Autodesk Fusion 360 part; units mm, degrees
note: some values were not read from the file. Set by a fixed rule: which sketch regions a step uses.
(part 3 of 20)
  spline S10 degree 5 poles (-7.9771, -12.1359) (-7.9772, -12.1359) (-7.9772, -12.136) (-7.9774, -12.1362) (-7.9776, -12.1365) (-7.9779, -12.137) (-7.9782, -12.1375) (-7.9786, -12.1381) (-7.979, -12.1388) (-7.9794, -12.1395) (-7.9799, -12.1403) (-7.9804, -12.1411) (-7.981, -12.1421) (-7.9816, -12.1431) (-7.9823, -12.1441) (-7.9829, -12.1452) (-7.9836, -12.1464) (-7.9844, -12.1477) (-7.9852, -12.149) (-7.986, -12.1504) (-7.9868, -12.1518) (-7.9877, -12.1533) (-7.9886, -12.1549) (-7.9896, -12.1565) (-7.9905, -12.1582) (-7.9915, -12.16) (-7.9926, -12.1618) (-7.9936, -12.1637) (-7.9947, -12.1656) (-7.9958, -12.1676) (-7.997, -12.1696) (-7.9982, -12.1718) (-7.9994, -12.1739) (-8.0006, -12.1762) (-8.0018, -12.1785) (-8.0031, -12.1808) (-8.0044, -12.1832) (-8.0057, -12.1857) (-8.0071, -12.1882) (-8.0084, -12.1908) (-8.0098, -12.1934) (-8.0113, -12.1961) (-8.0127, -12.1988) (-8.0142, -12.2016) (-8.0156, -12.2045) (-8.0171, -12.2074) (-8.0187, -12.2104) (-8.0202, -12.2134) (-8.0218, -12.2164) (-8.0233, -12.2196) (-8.0249, -12.2228) (-8.0265, -12.226) (-8.0282, -12.2293) (-8.0298, -12.2326) (-8.0315, -12.236) (-8.0332, -12.2395) (-8.0349, -12.243) (-8.0366, -12.2465) (-8.0383, -12.2501) (-8.0401, -12.2538) (-8.0419, -12.2575) (-8.0436, -12.2612) (-8.0454, -12.265) (-8.0472, -12.2689) (-8.0491, -12.2728) (-8.0509, -12.2768) (-8.0527, -12.2808) (-8.0546, -12.2848) (-8.0565, -12.289) (-8.0584, -12.2931) (-8.0603, -12.2973) (-8.0622, -12.3016) (-8.0641, -12.3059) (-8.066, -12.3102) (-8.068, -12.3146) (-8.0699, -12.3191) (-8.0719, -12.3236) (-8.0739, -12.3281) (-8.0759, -12.3327) (-8.0779, -12.3374) (-8.0799, -12.3421) (-8.0819, -12.3468) (-8.0839, -12.3516) (-8.0859, -12.3564) (-8.088, -12.3613) (-8.09, -12.3662) (-8.0921, -12.3712) (-8.0941, -12.3762) (-8.0962, -12.3813) (-8.0983, -12.3864) (-8.1004, -12.3915) (-8.1025, -12.3967) (-8.1046, -12.402) (-8.1067, -12.4073) (-8.1088, -12.4126) (-8.1109, -12.418) (-8.113, -12.4234) (-8.1151, -12.4289) (-8.1173, -12.4344) (-8.1194, -12.4399) (-8.1215, -12.4455) (-8.1237, -12.4512) (-8.1258, -12.4568) (-8.128, -12.4626) (-8.1302, -12.4683) (-8.1323, -12.4742) (-8.1345, -12.48) (-8.1366, -12.4859) (-8.1388, -12.4919) (-8.141, -12.4979) (-8.1432, -12.5039) (-8.1453, -12.51) (-8.1475, -12.5161) (-8.1497, -12.5222) (-8.1519, -12.5284) (-8.1541, -12.5347) (-8.1563, -12.5409) (-8.1584, -12.5473) (-8.1606, -12.5536) (-8.1628, -12.56) (-8.165, -12.5665) (-8.1672, -12.5729) (-8.1694, -12.5795) (-8.1716, -12.586) (-8.1738, -12.5926) (-8.176, -12.5993) (-8.1782, -12.606) (-8.1803, -12.6127) (-8.1825, -12.6195) (-8.1847, -12.6263) (-8.1869, -12.6331) (-8.1891, -12.64) (-8.1913, -12.6469) (-8.1935, -12.6539) (-8.1956, -12.6609) (-8.1978, -12.6679) (-8.2, -12.675) (-8.2022, -12.6821) (-8.2044, -12.6893) (-8.2065, -12.6965) (-8.2087, -12.7037) (-8.2109, -12.711) (-8.213, -12.7183) (-8.2152, -12.7256) (-8.2173, -12.733) (-8.2195, -12.7404) (-8.2216, -12.7479) (-8.2238, -12.7554) (-8.2259, -12.7629) (-8.2281, -12.7705) (-8.2302, -12.7781) (-8.2323, -12.7857) (-8.2345, -12.7934) (-8.2366, -12.8011) (-8.2387, -12.8089) (-8.2408, -12.8167) (-8.2429, -12.8245) (-8.245, -12.8324) (-8.2471, -12.8403) (-8.2492, -12.8482) (-8.2513, -12.8562) (-8.2534, -12.8642) (-8.2554, -12.8722) (-8.2575, -12.8803) (-8.2596, -12.8884) (-8.2616, -12.8966) (-8.2637, -12.9048) (-8.2657, -12.913) (-8.2678, -12.9212) (-8.2698, -12.9295) (-8.2718, -12.9379) (-8.2738, -12.9462) (-8.2759, -12.9546) (-8.2779, -12.963) (-8.2799, -12.9715) (-8.2818, -12.98) (-8.2838, -12.9885) (-8.2858, -12.9971) (-8.2878, -13.0057) (-8.2897, -13.0143) (-8.2917, -13.023) (-8.2936, -13.0317) (-8.2956, -13.0404) (-8.2975, -13.0492) (-8.2994, -13.058) (-8.3013, -13.0668) (-8.3032, -13.0757) (-8.3051, -13.0846) (-8.307, -13.0935) (-8.3089, -13.1025) (-8.3107, -13.1115) (-8.3126, -13.1205) (-8.3145, -13.1296) (-8.3163, -13.1386) (-8.3181, -13.1478) (-8.3199, -13.1569) (-8.3218, -13.1661) (-8.3236, -13.1753) (-8.3254, -13.1846) (-8.3271, -13.1939) (-8.3289, -13.2032) (-8.3307, -13.2125) (-8.3324, -13.2219) (-8.3342, -13.2313) (-8.3359, -13.2408) (-8.3376, -13.2503) (-8.3393, -13.2598) (-8.341, -13.2693) (-8.3427, -13.2789) (-8.3444, -13.2885) (-8.3461, -13.2981) (-8.3477, -13.3078) (-8.3494, -13.3174) (-8.351, -13.3272) (-8.3526, -13.3369) (-8.3542, -13.3467) (-8.3558, -13.3565) (-8.3574, -13.3663) (-8.359, -13.3762) (-8.3606, -13.3861) (-8.3621, -13.396) (-8.3637, -13.406) (-8.3652, -13.416) (-8.3667, -13.426) (-8.3682, -13.4361) (-8.3697, -13.4461) (-8.3712, -13.4563) (-8.3726, -13.4664) (-8.3741, -13.4766) (-8.3755, -13.4867) (-8.377, -13.497) (-8.3784, -13.5072) (-8.3798, -13.5175) (-8.3812, -13.5278) (-8.3826, -13.5382) (-8.3839, -13.5485) (-8.3853, -13.5589) (-8.3866, -13.5693) (-8.3879, -13.5798) (-8.3893, -13.5903) (-8.3906, -13.6008) (-8.3916, -13.6092) (-8.3924, -13.6155) (-8.3929, -13.6198) (-8.3931, -13.6219) knots 0 0 0 0 0 0 0.00416667 0.00833333 0.0125 0.01666667 0.02083333 0.025 0.02916667 0.03333333 0.0375 0.04166667 0.04583333 0.05 0.05416667 0.05833333 0.0625 0.06666667 0.07083333 0.075 0.07916667 0.08333333 0.0875 0.09166667 0.09583333 0.1 0.10416667 0.10833333 0.1125 0.11666667 0.12083333 0.125 0.12916667 0.13333333 0.1375 0.14166667 0.14583333 0.15 0.15416667 0.15833333 0.1625 0.16666667 0.17083333 0.175 0.17916667 0.18333333 0.1875 0.19166667 0.19583333 0.2 0.20416667 0.20833333 0.2125 0.21666667 0.22083333 0.225 0.22916667 0.23333333 0.2375 0.24166667 0.24583333 0.25 0.25416667 0.25833333 0.2625 0.26666667 0.27083333 0.275 0.27916667 0.28333333 0.2875 0.29166667 0.29583333 0.3 0.30416667 0.30833333 0.3125 0.31666667 0.32083333 0.325 0.32916667 0.33333333 0.3375 0.34166667 0.34583333 0.35 0.35416667 0.35833333 0.3625 0.36666667 0.37083333 0.375 0.37916667 0.38333333 0.3875 0.39166667 0.39583333 0.4 0.40416667 0.40833333 0.4125 0.41666667 0.42083333 0.425 0.42916667 0.43333333 0.4375 0.44166667 0.44583333 0.45 0.45416667 0.45833333 0.4625 0.46666667 0.47083333 0.475 0.47916667 0.48333333 0.4875 0.49166667 0.49583333 0.5 0.50416667 0.50833333 0.5125 0.51666667 0.52083333 0.525 0.52916667 0.53333333 0.5375 0.54166667 0.54583333 0.55 0.55416667 0.55833333 0.5625 0.56666667 0.57083333 0.575 0.57916667 0.58333333 0.5875 0.59166667 0.59583333 0.6 0.60416667 0.60833333 0.6125 0.61666667 0.62083333 0.625 0.62916667 0.63333333 0.6375 0.64166667 0.64583333 0.65 0.65416667 0.65833333 0.6625 0.66666667 0.67083333 0.675 0.67916667 0.68333333 0.6875 0.69166667 0.69583333 0.7 0.70416667 0.70833333 0.7125 0.71666667 0.72083333 0.725 0.72916667 0.73333333 0.7375 0.74166667 0.74583333 0.75 0.75416667 0.75833333 0.7625 0.76666667 0.77083333 0.775 0.77916667 0.78333333 0.7875 0.79166667 0.79583333 0.8 0.80416667 0.80833333 0.8125 0.81666667 0.82083333 0.825 0.82916667 0.83333333 0.8375 0.84166667 0.84583333 0.85 0.85416667 0.85833333 0.8625 0.86666667 0.87083333 0.875 0.87916667 0.88333333 0.8875 0.89166667 0.89583333 0.9 0.90416667 0.90833333 0.9125 0.91666667 0.92083333 0.925 0.92916667 0.93333333 0.9375 0.94166667 0.94583333 0.95 0.95416667 0.95833333 0.9625 0.96666667 0.97083333 0.975 0.97916667 0.98333333 0.9875 0.99166667 0.99583333 1 1 1 1 1 1
  arc A11 (-8.3931, -13.6219) -> (-7.6003, -14.0796) centre (0, 0) ccw
  spline S11 degree 5 poles (-7.6003, -14.0796) (-7.5986, -14.0783) (-7.5952, -14.0758) (-7.5901, -14.0719) (-7.5833, -14.0668) (-7.5749, -14.0604) (-7.5665, -14.0541) (-7.5581, -14.0477) (-7.5497, -14.0413) (-7.5414, -14.035) (-7.5331, -14.0286) (-7.5248, -14.0222) (-7.5166, -14.0159) (-7.5084, -14.0095) (-7.5002, -14.0032) (-7.4921, -13.9968) (-7.484, -13.9905) (-7.4759, -13.9841) (-7.4679, -13.9778) (-7.4599, -13.9714) (-7.4519, -13.9651) (-7.4439, -13.9588) (-7.436, -13.9525) (-7.4281, -13.9461) (-7.4203, -13.9398) (-7.4124, -13.9335) (-7.4046, -13.9272) (-7.3969, -13.9209) (-7.3892, -13.9146) (-7.3815, -13.9083) (-7.3738, -13.902) (-7.3662, -13.8958) (-7.3586, -13.8895) (-7.351, -13.8832) (-7.3435, -13.8769) (-7.336, -13.8707) (-7.3285, -13.8644) (-7.321, -13.8582) (-7.3136, -13.8519) (-7.3063, -13.8457) (-7.2989, -13.8395) (-7.2916, -13.8333) (-7.2843, -13.827) (-7.2771, -13.8208) (-7.2699, -13.8146) (-7.2627, -13.8084) (-7.2555, -13.8023) (-7.2484, -13.7961) (-7.2413, -13.7899) (-7.2343, -13.7837) (-7.2272, -13.7776) (-7.2203, -13.7714) (-7.2133, -13.7653) (-7.2064, -13.7592) (-7.1995, -13.753) (-7.1926, -13.7469) (-7.1858, -13.7408) (-7.179, -13.7347) (-7.1723, -13.7286) (-7.1655, -13.7226) (-7.1588, -13.7165) (-7.1522, -13.7104) (-7.1455, -13.7044) (-7.1389, -13.6983) (-7.1324, -13.6923) (-7.1259, -13.6863) (-7.1194, -13.6803) (-7.1129, -13.6743) (-7.1065, -13.6683) (-7.1001, -13.6623) (-7.0937, -13.6563) (-7.0874, -13.6504) (-7.0811, -13.6444) (-7.0748, -13.6385) (-7.0686, -13.6325) (-7.0624, -13.6266) (-7.0562, -13.6207) (-7.0501, -13.6148) (-7.044, -13.6089) (-7.0379, -13.6031) (-7.0319, -13.5972) (-7.0259, -13.5914) (-7.02, -13.5855) (-7.014, -13.5797) (-7.0081, -13.5739) (-7.0023, -13.5681) (-6.9965, -13.5624) (-6.9907, -13.5566) (-6.9849, -13.5508) (-6.9792, -13.5451) (-6.9735, -13.5394) (-6.9678, -13.5337) (-6.9622, -13.528) (-6.9566, -13.5223) (-6.9511, -13.5166) (-6.9455, -13.511) (-6.94, -13.5053) (-6.9346, -13.4997) (-6.9292, -13.4941) (-6.9238, -13.4885) (-6.9184, -13.4829) (-6.9131, -13.4774) (-6.9078, -13.4718) (-6.9026, -13.4663) (-6.8974, -13.4608) (-6.8922, -13.4553) (-6.8871, -13.4498) (-6.8819, -13.4444) (-6.8769, -13.4389) (-6.8718, -13.4335) (-6.8668, -13.4281) (-6.8618, -13.4227) (-6.8569, -13.4173) (-6.852, -13.412) (-6.8471, -13.4066) (-6.8423, -13.4013) (-6.8375, -13.396) (-6.8327, -13.3907) (-6.828, -13.3855) (-6.8233, -13.3802) (-6.8187, -13.375) (-6.814, -13.3698) (-6.8094, -13.3646) (-6.8049, -13.3595) (-6.8004, -13.3543) (-6.7959, -13.3492) (-6.7914, -13.3441) (-6.787, -13.339) (-6.7826, -13.334) (-6.7783, -13.329) (-6.774, -13.3239) (-6.7697, -13.319) (-6.7655, -13.314) (-6.7613, -13.309) (-6.7571, -13.3041) (-6.753, -13.2992) (-6.7489, -13.2944) (-6.7448, -13.2895) (-6.7408, -13.2847) (-6.7368, -13.2799) (-6.7328, -13.2751) (-6.7289, -13.2703) (-6.725, -13.2656) (-6.7212, -13.2609) (-6.7174, -13.2562) (-6.7136, -13.2516) (-6.7098, -13.2469) (-6.7061, -13.2423) (-6.7025, -13.2378) (-6.6988, -13.2332) (-6.6952, -13.2287) (-6.6917, -13.2242) (-6.6881, -13.2197) (-6.6846, -13.2153) (-6.6812, -13.2109) (-6.6778, -13.2065) (-6.6744, -13.2022) (-6.671, -13.1978) (-6.6677, -13.1935) (-6.6644, -13.1893) (-6.6612, -13.185) (-6.658, -13.1808) (-6.6548, -13.1767) (-6.6517, -13.1725) (-6.6486, -13.1684) (-6.6455, -13.1643) (-6.6425, -13.1603) (-6.6395, -13.1563) (-6.6366, -13.1523) (-6.6337, -13.1483) (-6.6308, -13.1444) (-6.628, -13.1405) (-6.6252, -13.1367) (-6.6224, -13.1328) (-6.6197, -13.1291) (-6.617, -13.1253) (-6.6143, -13.1216) (-6.6117, -13.1179) (-6.6091, -13.1143) (-6.6065, -13.1107) (-6.604, -13.1071) (-6.6016, -13.1036) (-6.5991, -13.1001) (-6.5967, -13.0966) (-6.5944, -13.0932) (-6.592, -13.0898) (-6.5897, -13.0865) (-6.5875, -13.0832) (-6.5853, -13.0799) (-6.5831, -13.0767) (-6.581, -13.0735) (-6.5788, -13.0703) (-6.5768, -13.0672) (-6.5747, -13.0642) (-6.5728, -13.0612) (-6.5708, -13.0582) (-6.5689, -13.0553) (-6.567, -13.0524) (-6.5651, -13.0495) (-6.5633, -13.0467) (-6.5616, -13.044) (-6.5598, -13.0413) (-6.5581, -13.0386) (-6.5565, -13.036) (-6.5549, -13.0334) (-6.5533, -13.0309) (-6.5517, -13.0284) (-6.5502, -13.026) (-6.5488, -13.0236) (-6.5473, -13.0213) (-6.5459, -13.019) (-6.5446, -13.0168) (-6.5433, -13.0146) (-6.542, -13.0125) (-6.5407, -13.0104) (-6.5395, -13.0084) (-6.5384, -13.0064) (-6.5372, -13.0045) (-6.5361, -13.0027) (-6.5351, -13.0009) (-6.5341, -12.9991) (-6.5331, -12.9974) (-6.5321, -12.9958) (-6.5312, -12.9942) (-6.5304, -12.9927) (-6.5295, -12.9913) (-6.5288, -12.9899) (-6.528, -12.9885) (-6.5273, -12.9873) (-6.5266, -12.986) (-6.526, -12.9849) (-6.5254, -12.9838) (-6.5248, -12.9828) (-6.5243, -12.9818) (-6.5238, -12.9809) (-6.5234, -12.9801) (-6.523, -12.9794) (-6.5226, -12.9787) (-6.5223, -12.9781) (-6.522, -12.9775) (-6.5218, -12.977) (-6.5216, -12.9767) (-6.5215, -12.9765) (-6.5214, -12.9764) (-6.5214, -12.9763) knots -1 -1 -1 -1 -1 -1 -0.99583333 -0.99166667 -0.9875 -0.98333333 -0.97916667 -0.975 -0.97083333 -0.96666667 -0.9625 -0.95833333 -0.95416667 -0.95 -0.94583333 -0.94166667 -0.9375 -0.93333333 -0.92916667 -0.925 -0.92083333 -0.91666667 -0.9125 -0.90833333 -0.90416667 -0.9 -0.89583333 -0.89166667 -0.8875 -0.88333333 -0.87916667 -0.875 -0.87083333 -0.86666667 -0.8625 -0.85833333 -0.85416667 -0.85 -0.84583333 -0.84166667 -0.8375 -0.83333333 -0.82916667 -0.825 -0.82083333 -0.81666667 -0.8125 -0.80833333 -0.80416667 -0.8 -0.79583333 -0.79166667 -0.7875 -0.78333333 -0.77916667 -0.775 -0.77083333 -0.76666667 -0.7625 -0.75833333 -0.75416667 -0.75 -0.74583333 -0.74166667 -0.7375 -0.73333333 -0.72916667 -0.725 -0.72083333 -0.71666667 -0.7125 -0.70833333 -0.70416667 -0.7 -0.69583333 -0.69166667 -0.6875 -0.68333333 -0.67916667 -0.675 -0.67083333 -0.66666667 -0.6625 -0.65833333 -0.65416667 -0.65 -0.64583333 -0.64166667 -0.6375 -0.63333333 -0.62916667 -0.625 -0.62083333 -0.61666667 -0.6125 -0.60833333 -0.60416667 -0.6 -0.59583333 -0.59166667 -0.5875 -0.58333333 -0.57916667 -0.575 -0.57083333 -0.56666667 -0.5625 -0.55833333 -0.55416667 -0.55 -0.54583333 -0.54166667 -0.5375 -0.53333333 -0.52916667 -0.525 -0.52083333 -0.51666667 -0.5125 -0.50833333 -0.50416667 -0.5 -0.49583333 -0.49166667 -0.4875 -0.48333333 -0.47916667 -0.475 -0.47083333 -0.46666667 -0.4625 -0.45833333 -0.45416667 -0.45 -0.44583333 -0.44166667 -0.4375 -0.43333333 -0.42916667 -0.425 -0.42083333 -0.41666667 -0.4125 -0.40833333 -0.40416667 -0.4 -0.39583333 -0.39166667 -0.3875 -0.38333333 -0.37916667 -0.375 -0.37083333 -0.36666667 -0.3625 -0.35833333 -0.35416667 -0.35 -0.34583333 -0.34166667 -0.3375 -0.33333333 -0.32916667 -0.325 -0.32083333 -0.31666667 -0.3125 -0.30833333 -0.30416667 -0.3 -0.29583333 -0.29166667 -0.2875 -0.28333333 -0.27916667 -0.275 -0.27083333 -0.26666667 -0.2625 -0.25833333 -0.25416667 -0.25 -0.24583333 -0.24166667 -0.2375 -0.23333333 -0.22916667 -0.225 -0.22083333 -0.21666667 -0.2125 -0.20833333 -0.20416667 -0.2 -0.19583333 -0.19166667 -0.1875 -0.18333333 -0.17916667 -0.175 -0.17083333 -0.16666667 -0.1625 -0.15833333 -0.15416667 -0.15 -0.14583333 -0.14166667 -0.1375 -0.13333333 -0.12916667 -0.125 -0.12083333 -0.11666667 -0.1125 -0.10833333 -0.10416667 -0.1 -0.09583333 -0.09166667 -0.0875 -0.08333333 -0.07916667 -0.075 -0.07083333 -0.06666667 -0.0625 -0.05833333 -0.05416667 -0.05 -0.04583333 -0.04166667 -0.0375 -0.03333333 -0.02916667 -0.025 -0.02083333 -0.01666667 -0.0125 -0.00833333 -0.00416667 0 0 0 0 0 0
  line L22 (-6.5214, -12.9763) -> (-6.5211, -12.9757)
  line L23 (-6.5211, -12.9757) -> (-6.1743, -12.2858)
  arc A12 (-6.1743, -12.2858) -> (-4.9987, -12.8092) centre (0, 0) ccw
  line L24 (-4.9987, -12.8092) -> (-5.2794, -13.5286)
  line L25 (-5.2794, -13.5286) -> (-5.2796, -13.5292)
  spline S12 degree 5 poles (-5.2796, -13.5292) (-5.2796, -13.5293) (-5.2797, -13.5294) (-5.2798, -13.5296) (-5.2799, -13.53) (-5.2801, -13.5305) (-5.2803, -13.531) (-5.2805, -13.5317) (-5.2808, -13.5324) (-5.2811, -13.5332) (-5.2814, -13.5341) (-5.2818, -13.5351) (-5.2821, -13.5361) (-5.2825, -13.5372) (-5.2829, -13.5383) (-5.2833, -13.5396) (-5.2838, -13.5409) (-5.2843, -13.5423) (-5.2848, -13.5437) (-5.2853, -13.5452) (-5.2858, -13.5468) (-5.2863, -13.5485) (-5.2869, -13.5502) (-5.2875, -13.552) (-5.2881, -13.5539) (-5.2887, -13.5558) (-5.2893, -13.5578) (-5.29, -13.5598) (-5.2907, -13.5619) (-5.2913, -13.5641) (-5.292, -13.5664) (-5.2927, -13.5687) (-5.2935, -13.5711) (-5.2942, -13.5735) (-5.2949, -13.576) (-5.2957, -13.5786) (-5.2965, -13.5812) (-5.2972, -13.5839) (-5.298, -13.5866) (-5.2988, -13.5894) (-5.2997, -13.5923) (-5.3005, -13.5952) (-5.3013, -13.5982) (-5.3022, -13.6012) (-5.303, -13.6043) (-5.3039, -13.6075) (-5.3047, -13.6107) (-5.3056, -13.614) (-5.3065, -13.6173) (-5.3074, -13.6207) (-5.3083, -13.6241) (-5.3092, -13.6276) (-5.3101, -13.6312) (-5.3111, -13.6348) (-5.312, -13.6385) (-5.3129, -13.6422) (-5.3138, -13.646) (-5.3148, -13.6498) (-5.3157, -13.6537) (-5.3167, -13.6576) (-5.3176, -13.6616) (-5.3186, -13.6657) (-5.3196, -13.6698) (-5.3205, -13.6739) (-5.3215, -13.6781) (-5.3225, -13.6824) (-5.3235, -13.6867) (-5.3244, -13.691) (-5.3254, -13.6954) (-5.3264, -13.6999) (-5.3274, -13.7044) (-5.3284, -13.709) (-5.3293, -13.7136) (-5.3303, -13.7183) (-5.3313, -13.723) (-5.3323, -13.7277) (-5.3333, -13.7325) (-5.3343, -13.7374) (-5.3353, -13.7423) (-5.3363, -13.7473) (-5.3372, -13.7523) (-5.3382, -13.7573) (-5.3392, -13.7624) (-5.3402, -13.7676) (-5.3412, -13.7728) (-5.3422, -13.778) (-5.3431, -13.7833) (-5.3441, -13.7886) (-5.3451, -13.794) (-5.3461, -13.7994) (-5.347, -13.8049) (-5.348, -13.8104) (-5.3489, -13.816) (-5.3499, -13.8216) (-5.3509, -13.8273) (-5.3518, -13.833) (-5.3528, -13.8387) (-5.3537, -13.8445) (-5.3546, -13.8503) (-5.3556, -13.8562) (-5.3565, -13.8621) (-5.3574, -13.8681) (-5.3583, -13.8741) (-5.3593, -13.8801) (-5.3602, -13.8862) (-5.3611, -13.8924) (-5.362, -13.8986) (-5.3629, -13.9048) (-5.3638, -13.911) (-5.3646, -13.9173) (-5.3655, -13.9237) (-5.3664, -13.9301) (-5.3672, -13.9365) (-5.3681, -13.943) (-5.3689, -13.9495) (-5.3698, -13.9561) (-5.3706, -13.9627) (-5.3714, -13.9693) (-5.3723, -13.976) (-5.3731, -13.9827) (-5.3739, -13.9895) (-5.3747, -13.9963) (-5.3755, -14.0031) (-5.3762, -14.01) (-5.377, -14.0169) (-5.3778, -14.0238) (-5.3785, -14.0308) (-5.3793, -14.0379) (-5.38, -14.0449) (-5.3807, -14.0521) (-5.3814, -14.0592) (-5.3821, -14.0664) (-5.3828, -14.0736) (-5.3835, -14.0809) (-5.3842, -14.0882) (-5.3849, -14.0955) (-5.3855, -14.1029) (-5.3862, -14.1103) (-5.3868, -14.1178) (-5.3874, -14.1253) (-5.3881, -14.1328) (-5.3887, -14.1403) (-5.3893, -14.1479) (-5.3899, -14.1556) (-5.3904, -14.1632) (-5.391, -14.171) (-5.3915, -14.1787) (-5.3921, -14.1865) (-5.3926, -14.1943) (-5.3931, -14.2021) (-5.3936, -14.21) (-5.3941, -14.2179) (-5.3946, -14.2259) (-5.3951, -14.2339) (-5.3955, -14.2419) (-5.396, -14.25) (-5.3964, -14.2581) (-5.3968, -14.2662) (-5.3973, -14.2744) (-5.3976, -14.2826) (-5.398, -14.2908) (-5.3984, -14.2991) (-5.3988, -14.3074) (-5.3991, -14.3157) (-5.3994, -14.3241) (-5.3998, -14.3325) (-5.4001, -14.3409) (-5.4003, -14.3493) (-5.4006, -14.3578) (-5.4009, -14.3664) (-5.4011, -14.3749) (-5.4014, -14.3835) (-5.4016, -14.3922) (-5.4018, -14.4008) (-5.402, -14.4095) (-5.4022, -14.4182) (-5.4023, -14.427) (-5.4025, -14.4358) (-5.4026, -14.4446) (-5.4028, -14.4535) (-5.4029, -14.4623) (-5.403, -14.4712) (-5.403, -14.4802) (-5.4031, -14.4892) (-5.4031, -14.4982) (-5.4032, -14.5072) (-5.4032, -14.5163) (-5.4032, -14.5254) (-5.4032, -14.5345) (-5.4032, -14.5437) (-5.4031, -14.5528) (-5.4031, -14.5621) (-5.403, -14.5713) (-5.4029, -14.5806) (-5.4028, -14.5899) (-5.4027, -14.5992) (-5.4025, -14.6086) (-5.4024, -14.618) (-5.4022, -14.6274) (-5.402, -14.6369) (-5.4018, -14.6464) (-5.4016, -14.6559) (-5.4013, -14.6654) (-5.4011, -14.675) (-5.4008, -14.6846) (-5.4005, -14.6942) (-5.4002, -14.7038) (-5.3999, -14.7135) (-5.3996, -14.7232) (-5.3992, -14.733) (-5.3988, -14.7427) (-5.3985, -14.7525) (-5.3981, -14.7624) (-5.3976, -14.7722) (-5.3972, -14.7821) (-5.3967, -14.792) (-5.3963, -14.8019) (-5.3958, -14.8119) (-5.3953, -14.8218) (-5.3947, -14.8319) (-5.3942, -14.8419) (-5.3936, -14.852) (-5.393, -14.862) (-5.3924, -14.8722) (-5.3918, -14.8823) (-5.3912, -14.8925) (-5.3905, -14.9027) (-5.3899, -14.9129) (-5.3892, -14.9231) (-5.3885, -14.9334) (-5.3877, -14.9437) (-5.387, -14.954) (-5.3862, -14.9644) (-5.3854, -14.9747) (-5.3846, -14.9851) (-5.3838, -14.9956) (-5.383, -15.006) (-5.3821, -15.0165) (-5.3813, -15.027) (-5.3804, -15.0375) (-5.3794, -15.0481) (-5.3787, -15.0565) (-5.3781, -15.0629) (-5.3777, -15.0671) (-5.3776, -15.0692) knots 0 0 0 0 0 0 0.00416667 0.00833333 0.0125 0.01666667 0.02083333 0.025 0.02916667 0.03333333 0.0375 0.04166667 0.04583333 0.05 0.05416667 0.05833333 0.0625 0.06666667 0.07083333 0.075 0.07916667 0.08333333 0.0875 0.09166667 0.09583333 0.1 0.10416667 0.10833333 0.1125 0.11666667 0.12083333 0.125 0.12916667 0.13333333 0.1375 0.14166667 0.14583333 0.15 0.15416667 0.15833333 0.1625 0.16666667 0.17083333 0.175 0.17916667 0.18333333 0.1875 0.19166667 0.19583333 0.2 0.20416667 0.20833333 0.2125 0.21666667 0.22083333 0.225 0.22916667 0.23333333 0.2375 0.24166667 0.24583333 0.25 0.25416667 0.25833333 0.2625 0.26666667 0.27083333 0.275 0.27916667 0.28333333 0.2875 0.29166667 0.29583333 0.3 0.30416667 0.30833333 0.3125 0.31666667 0.32083333 0.325 0.32916667 0.33333333 0.3375 0.34166667 0.34583333 0.35 0.35416667 0.35833333 0.3625 0.36666667 0.37083333 0.375 0.37916667 0.38333333 0.3875 0.39166667 0.39583333 0.4 0.40416667 0.40833333 0.4125 0.41666667 0.42083333 0.425 0.42916667 0.43333333 0.4375 0.44166667 0.44583333 0.45 0.45416667 0.45833333 0.4625 0.46666667 0.47083333 0.475 0.47916667 0.48333333 0.4875 0.49166667 0.49583333 0.5 0.50416667 0.50833333 0.5125 0.51666667 0.52083333 0.525 0.52916667 0.53333333 0.5375 0.54166667 0.54583333 0.55 0.55416667 0.55833333 0.5625 0.56666667 0.57083333 0.575 0.57916667 0.58333333 0.5875 0.59166667 0.59583333 0.6 0.60416667 0.60833333 0.6125 0.61666667 0.62083333 0.625 0.62916667 0.63333333 0.6375 0.64166667 0.64583333 0.65 0.65416667 0.65833333 0.6625 0.66666667 0.67083333 0.675 0.67916667 0.68333333 0.6875 0.69166667 0.69583333 0.7 0.70416667 0.70833333 0.7125 0.71666667 0.72083333 0.725 0.72916667 0.73333333 0.7375 0.74166667 0.74583333 0.75 0.75416667 0.75833333 0.7625 0.76666667 0.77083333 0.775 0.77916667 0.78333333 0.7875 0.79166667 0.79583333 0.8 0.80416667 0.80833333 0.8125 0.81666667 0.82083333 0.825 0.82916667 0.83333333 0.8375 0.84166667 0.84583333 0.85 0.85416667 0.85833333 0.8625 0.86666667 0.87083333 0.875 0.87916667 0.88333333 0.8875 0.89166667 0.89583333 0.9 0.90416667 0.90833333 0.9125 0.91666667 0.92083333 0.925 0.92916667 0.93333333 0.9375 0.94166667 0.94583333 0.95 0.95416667 0.95833333 0.9625 0.96666667 0.97083333 0.975 0.97916667 0.98333333 0.9875 0.99166667 0.99583333 1 1 1 1 1 1
  arc A13 (-5.3776, -15.0692) -> (-4.5069, -15.3521) centre (0, 0) ccw
  spline S13 degree 5 poles (-4.5069, -15.3521) (-4.5055, -15.3505) (-4.5027, -15.3473) (-4.4985, -15.3425) (-4.493, -15.3361) (-4.486, -15.3281) (-4.4791, -15.3201) (-4.4722, -15.3121) (-4.4654, -15.3042) (-4.4586, -15.2962) (-4.4518, -15.2883) (-4.445, -15.2803) (-4.4383, -15.2724) (-4.4316, -15.2645) (-4.4249, -15.2565) (-4.4183, -15.2486) (-4.4117, -15.2407) (-4.4051, -15.2329) (-4.3985, -15.225) (-4.392, -15.2171) (-4.3855, -15.2093) (-4.3791, -15.2014) (-4.3726, -15.1936) (-4.3662, -15.1858) (-4.3599, -15.178) (-4.3535, -15.1702) (-4.3472, -15.1624) (-4.3409, -15.1546) (-4.3347, -15.1468) (-4.3285, -15.1391) (-4.3223, -15.1313) (-4.3161, -15.1236) (-4.31, -15.1159) (-4.3039, -15.1082) (-4.2978, -15.1005) (-4.2918, -15.0928) (-4.2858, -15.0851) (-4.2798, -15.0775) (-4.2738, -15.0698) (-4.2679, -15.0622) (-4.262, -15.0546) (-4.2562, -15.047) (-4.2503, -15.0394) (-4.2445, -15.0318) (-4.2388, -15.0242) (-4.233, -15.0167) (-4.2273, -15.0092) (-4.2216, -15.0016) (-4.216, -14.9941) (-4.2104, -14.9866) (-4.2048, -14.9791) (-4.1992, -14.9717) (-4.1937, -14.9642) (-4.1882, -14.9568) (-4.1827, -14.9494) (-4.1773, -14.942) (-4.1719, -14.9346) (-4.1665, -14.9272) (-4.1612, -14.9198) (-4.1559, -14.9125) (-4.1506, -14.9052) (-4.1453, -14.8978) (-4.1401, -14.8905) (-4.1349, -14.8833) (-4.1297, -14.876) (-4.1246, -14.8687) (-4.1195, -14.8615) (-4.1144, -14.8543) (-4.1094, -14.8471) (-4.1044, -14.8399) (-4.0994, -14.8328) (-4.0944, -14.8256) (-4.0895, -14.8185) (-4.0846, -14.8114) (-4.0798, -14.8043) (-4.0749, -14.7972) (-4.0701, -14.7901) (-4.0654, -14.7831) (-4.0606, -14.7761) (-4.0559, -14.7691) (-4.0512, -14.7621) (-4.0466, -14.7551) (-4.042, -14.7482) (-4.0374, -14.7413) (-4.0328, -14.7344) (-4.0283, -14.7275) (-4.0238, -14.7206) (-4.0193, -14.7138) (-4.0149, -14.707) (-4.0105, -14.7002) (-4.0061, -14.6934) (-4.0018, -14.6866) (-3.9974, -14.6799) (-3.9932, -14.6731) (-3.9889, -14.6665) (-3.9847, -14.6598) (-3.9805, -14.6531) (-3.9763, -14.6465) (-3.9722, -14.6399) (-3.9681, -14.6333) (-3.964, -14.6267) (-3.96, -14.6202) (-3.9559, -14.6137) (-3.952, -14.6072) (-3.948, -14.6007) (-3.9441, -14.5942) (-3.9402, -14.5878) (-3.9363, -14.5814) (-3.9325, -14.575) (-3.9287, -14.5687) (-3.9249, -14.5623) (-3.9212, -14.556) (-3.9175, -14.5497) (-3.9138, -14.5435) (-3.9101, -14.5373) (-3.9065, -14.5311) (-3.9029, -14.5249) (-3.8993, -14.5187) (-3.8958, -14.5126) (-3.8923, -14.5065) (-3.8888, -14.5004) (-3.8854, -14.4944) (-3.882, -14.4883) (-3.8786, -14.4824) (-3.8752, -14.4764) (-3.8719, -14.4704) (-3.8686, -14.4645) (-3.8654, -14.4587) (-3.8621, -14.4528) (-3.8589, -14.447) (-3.8558, -14.4412) (-3.8526, -14.4354) (-3.8495, -14.4297) (-3.8464, -14.424) (-3.8434, -14.4183) (-3.8403, -14.4126) (-3.8373, -14.407) (-3.8344, -14.4014) (-3.8314, -14.3959) (-3.8285, -14.3903) (-3.8257, -14.3848) (-3.8228, -14.3794) (-3.82, -14.3739) (-3.8172, -14.3685) (-3.8144, -14.3632) (-3.8117, -14.3578) (-3.809, -14.3525) (-3.8063, -14.3473) (-3.8037, -14.342) (-3.8011, -14.3368) (-3.7985, -14.3316) (-3.796, -14.3265) (-3.7934, -14.3214) (-3.791, -14.3163) (-3.7885, -14.3113) (-3.7861, -14.3063) (-3.7836, -14.3013) (-3.7813, -14.2964) (-3.7789, -14.2915) (-3.7766, -14.2867) (-3.7743, -14.2819) (-3.7721, -14.2771) (-3.7698, -14.2723) (-3.7676, -14.2676) (-3.7655, -14.263) (-3.7633, -14.2583) (-3.7612, -14.2537) (-3.7591, -14.2492) (-3.7571, -14.2447) (-3.755, -14.2402) (-3.753, -14.2358) (-3.7511, -14.2314) (-3.7491, -14.227) (-3.7472, -14.2227) (-3.7453, -14.2185) (-3.7435, -14.2142) (-3.7416, -14.21) (-3.7398, -14.2059) (-3.7381, -14.2018) (-3.7363, -14.1977) (-3.7346, -14.1937) (-3.7329, -14.1898) (-3.7313, -14.1858) (-3.7296, -14.1819) (-3.728, -14.1781) (-3.7265, -14.1743) (-3.7249, -14.1706) (-3.7234, -14.1669) (-3.7219, -14.1632) (-3.7204, -14.1596) (-3.719, -14.1561) (-3.7176, -14.1525) (-3.7162, -14.1491) (-3.7149, -14.1457) (-3.7136, -14.1423) (-3.7123, -14.139) (-3.711, -14.1357) (-3.7097, -14.1325) (-3.7085, -14.1293) (-3.7073, -14.1262) (-3.7062, -14.1232) (-3.7051, -14.1202) (-3.704, -14.1172) (-3.7029, -14.1143) (-3.7018, -14.1114) (-3.7008, -14.1086) (-3.6998, -14.1059) (-3.6988, -14.1032) (-3.6979, -14.1006) (-3.697, -14.098) (-3.6961, -14.0955) (-3.6952, -14.093) (-3.6944, -14.0906) (-3.6936, -14.0883) (-3.6928, -14.086) (-3.692, -14.0838) (-3.6913, -14.0816) (-3.6906, -14.0795) (-3.6899, -14.0775) (-3.6892, -14.0755) (-3.6886, -14.0736) (-3.688, -14.0717) (-3.6874, -14.0699) (-3.6869, -14.0682) (-3.6863, -14.0665) (-3.6858, -14.0649) (-3.6853, -14.0634) (-3.6849, -14.0619) (-3.6845, -14.0606) (-3.6841, -14.0592) (-3.6837, -14.058) (-3.6833, -14.0568) (-3.683, -14.0557) (-3.6827, -14.0546) (-3.6824, -14.0537) (-3.6821, -14.0528) (-3.6819, -14.0519) (-3.6817, -14.0512) (-3.6815, -14.0505) (-3.6813, -14.0499) (-3.6812, -14.0494) (-3.6811, -14.0491) (-3.681, -14.0488) (-3.681, -14.0487) (-3.681, -14.0486) knots -1 -1 -1 -1 -1 -1 -0.99583333 -0.99166667 -0.9875 -0.98333333 -0.97916667 -0.975 -0.97083333 -0.96666667 -0.9625 -0.95833333 -0.95416667 -0.95 -0.94583333 -0.94166667 -0.9375 -0.93333333 -0.92916667 -0.925 -0.92083333 -0.91666667 -0.9125 -0.90833333 -0.90416667 -0.9 -0.89583333 -0.89166667 -0.8875 -0.88333333 -0.87916667 -0.875 -0.87083333 -0.86666667 -0.8625 -0.85833333 -0.85416667 -0.85 -0.84583333 -0.84166667 -0.8375 -0.83333333 -0.82916667 -0.825 -0.82083333 -0.81666667 -0.8125 -0.80833333 -0.80416667 -0.8 -0.79583333 -0.79166667 -0.7875 -0.78333333 -0.77916667 -0.775 -0.77083333 -0.76666667 -0.7625 -0.75833333 -0.75416667 -0.75 -0.74583333 -0.74166667 -0.7375 -0.73333333 -0.72916667 -0.725 -0.72083333 -0.71666667 -0.7125 -0.70833333 -0.70416667 -0.7 -0.69583333 -0.69166667 -0.6875 -0.68333333 -0.67916667 -0.675 -0.67083333 -0.66666667 -0.6625 -0.65833333 -0.65416667 -0.65 -0.64583333 -0.64166667 -0.6375 -0.63333333 -0.62916667 -0.625 -0.62083333 -0.61666667 -0.6125 -0.60833333 -0.60416667 -0.6 -0.59583333 -0.59166667 -0.5875 -0.58333333 -0.57916667 -0.575 -0.57083333 -0.56666667 -0.5625 -0.55833333 -0.55416667 -0.55 -0.54583333 -0.54166667 -0.5375 -0.53333333 -0.52916667 -0.525 -0.52083333 -0.51666667 -0.5125 -0.50833333 -0.50416667 -0.5 -0.49583333 -0.49166667 -0.4875 -0.48333333 -0.47916667 -0.475 -0.47083333 -0.46666667 -0.4625 -0.45833333 -0.45416667 -0.45 -0.44583333 -0.44166667 -0.4375 -0.43333333 -0.42916667 -0.425 -0.42083333 -0.41666667 -0.4125 -0.40833333 -0.40416667 -0.4 -0.39583333 -0.39166667 -0.3875 -0.38333333 -0.37916667 -0.375 -0.37083333 -0.36666667 -0.3625 -0.35833333 -0.35416667 -0.35 -0.34583333 -0.34166667 -0.3375 -0.33333333 -0.32916667 -0.325 -0.32083333 -0.31666667 -0.3125 -0.30833333 -0.30416667 -0.3 -0.29583333 -0.29166667 -0.2875 -0.28333333 -0.27916667 -0.275 -0.27083333 -0.26666667 -0.2625 -0.25833333 -0.25416667 -0.25 -0.24583333 -0.24166667 -0.2375 -0.23333333 -0.22916667 -0.225 -0.22083333 -0.21666667 -0.2125 -0.20833333 -0.20416667 -0.2 -0.19583333 -0.19166667 -0.1875 -0.18333333 -0.17916667 -0.175 -0.17083333 -0.16666667 -0.1625 -0.15833333 -0.15416667 -0.15 -0.14583333 -0.14166667 -0.1375 -0.13333333 -0.12916667 -0.125 -0.12083333 -0.11666667 -0.1125 -0.10833333 -0.10416667 -0.1 -0.09583333 -0.09166667 -0.0875 -0.08333333 -0.07916667 -0.075 -0.07083333 -0.06666667 -0.0625 -0.05833333 -0.05416667 -0.05 -0.04583333 -0.04166667 -0.0375 -0.03333333 -0.02916667 -0.025 -0.02083333 -0.01666667 -0.0125 -0.00833333 -0.00416667 0 0 0 0 0 0
  line L26 (-3.681, -14.0486) -> (-3.6808, -14.048)
  line L27 (-3.6808, -14.048) -> (-3.4851, -13.301)
  arc A14 (-3.4851, -13.301) -> (-2.2262, -13.5686) centre (0, 0) ccw
  line L28 (-2.2262, -13.5686) -> (-2.3513, -14.3306)
  line L29 (-2.3513, -14.3306) -> (-2.3514, -14.3312)
  spline S14 degree 5 poles (-2.3514, -14.3312) (-2.3514, -14.3313) (-2.3514, -14.3314) (-2.3514, -14.3317) (-2.3515, -14.332) (-2.3516, -14.3326) (-2.3517, -14.3332) (-2.3518, -14.3339) (-2.3519, -14.3346) (-2.352, -14.3355) (-2.3521, -14.3364) (-2.3522, -14.3374) (-2.3524, -14.3385) (-2.3525, -14.3397) (-2.3527, -14.3409) (-2.3529, -14.3422) (-2.353, -14.3436) (-2.3532, -14.345) (-2.3534, -14.3465) (-2.3536, -14.3481) (-2.3537, -14.3498) (-2.3539, -14.3515) (-2.3541, -14.3533) (-2.3543, -14.3552) (-2.3545, -14.3571) (-2.3547, -14.3591) (-2.3549, -14.3612) (-2.3551, -14.3634) (-2.3554, -14.3656) (-2.3556, -14.3679) (-2.3558, -14.3702) (-2.356, -14.3726) (-2.3562, -14.3751) (-2.3564, -14.3776) (-2.3566, -14.3802) (-2.3568, -14.3829) (-2.357, -14.3856) (-2.3572, -14.3884) (-2.3575, -14.3912) (-2.3577, -14.3941) (-2.3579, -14.3971) (-2.3581, -14.4001) (-2.3583, -14.4032) (-2.3584, -14.4064) (-2.3586, -14.4096) (-2.3588, -14.4129) (-2.359, -14.4162) (-2.3592, -14.4196) (-2.3594, -14.423) (-2.3595, -14.4265) (-2.3597, -14.4301) (-2.3599, -14.4337) (-2.36, -14.4374) (-2.3602, -14.4411) (-2.3603, -14.4449) (-2.3604, -14.4487) (-2.3606, -14.4526) (-2.3607, -14.4565) (-2.3608, -14.4605) (-2.3609, -14.4646) (-2.361, -14.4687) (-2.3611, -14.4728) (-2.3612, -14.477) (-2.3613, -14.4813) (-2.3614, -14.4856) (-2.3614, -14.49) (-2.3615, -14.4944) (-2.3616, -14.4989) (-2.3616, -14.5034) (-2.3616, -14.5079) (-2.3616, -14.5126) (-2.3617, -14.5172) (-2.3617, -14.5219) (-2.3617, -14.5267) (-2.3617, -14.5315) (-2.3616, -14.5364) (-2.3616, -14.5413) (-2.3616, -14.5463) (-2.3615, -14.5513) (-2.3614, -14.5563) (-2.3614, -14.5614) (-2.3613, -14.5666) (-2.3612, -14.5718) (-2.3611, -14.577) (-2.3609, -14.5823) (-2.3608, -14.5876) (-2.3607, -14.593) (-2.3605, -14.5984) (-2.3603, -14.6039) (-2.3602, -14.6094) (-2.36, -14.6149) (-2.3598, -14.6205) (-2.3596, -14.6262) (-2.3593, -14.6319) (-2.3591, -14.6376) (-2.3588, -14.6434) (-2.3586, -14.6492) (-2.3583, -14.655) (-2.358, -14.6609) (-2.3577, -14.6669) (-2.3574, -14.6729) (-2.357, -14.6789) (-2.3567, -14.685) (-2.3563, -14.6911) (-2.3559, -14.6972) (-2.3555, -14.7034) (-2.3551, -14.7097) (-2.3547, -14.7159) (-2.3543, -14.7222) (-2.3538, -14.7286) (-2.3534, -14.735) (-2.3529, -14.7414) (-2.3524, -14.7479) (-2.3519, -14.7544) (-2.3513, -14.7609) (-2.3508, -14.7675) (-2.3503, -14.7742) (-2.3497, -14.7808) (-2.3491, -14.7875) (-2.3485, -14.7943) (-2.3479, -14.801) (-2.3472, -14.8079) (-2.3466, -14.8147) (-2.3459, -14.8216) (-2.3452, -14.8285) (-2.3445, -14.8355) (-2.3438, -14.8425) (-2.3431, -14.8495) (-2.3423, -14.8566) (-2.3416, -14.8637) (-2.3408, -14.8708) (-2.34, -14.878) (-2.3391, -14.8852) (-2.3383, -14.8925) (-2.3375, -14.8998) (-2.3366, -14.9071) (-2.3357, -14.9144) (-2.3348, -14.9218) (-2.3339, -14.9292) (-2.3329, -14.9367) (-2.332, -14.9442) (-2.331, -14.9517) (-2.33, -14.9593) (-2.329, -14.9669) (-2.3279, -14.9745) (-2.3269, -14.9821) (-2.3258, -14.9898) (-2.3247, -14.9975) (-2.3236, -15.0053) (-2.3225, -15.0131) (-2.3213, -15.0209) (-2.3202, -15.0288) (-2.319, -15.0366) (-2.3178, -15.0445) (-2.3166, -15.0525) (-2.3153, -15.0605) (-2.3141, -15.0685) (-2.3128, -15.0765) (-2.3115, -15.0846) (-2.3102, -15.0927) (-2.3088, -15.1008) (-2.3075, -15.109) (-2.3061, -15.1172) (-2.3047, -15.1254) (-2.3033, -15.1336) (-2.3019, -15.1419) (-2.3004, -15.1502) (-2.2989, -15.1586) (-2.2974, -15.1669) (-2.2959, -15.1753) (-2.2944, -15.1838) (-2.2928, -15.1922) (-2.2913, -15.2007) (-2.2897, -15.2092) (-2.288, -15.2178) (-2.2864, -15.2263) (-2.2847, -15.2349) (-2.2831, -15.2436) (-2.2814, -15.2522) (-2.2796, -15.2609) (-2.2779, -15.2696) (-2.2761, -15.2784) (-2.2744, -15.2871) (-2.2726, -15.2959) (-2.2707, -15.3047) (-2.2689, -15.3136) (-2.267, -15.3224) (-2.2651, -15.3313) (-2.2632, -15.3403) (-2.2613, -15.3492) (-2.2593, -15.3582) (-2.2574, -15.3672) (-2.2554, -15.3762) (-2.2533, -15.3853) (-2.2513, -15.3944) (-2.2492, -15.4035) (-2.2472, -15.4126) (-2.2451, -15.4218) (-2.2429, -15.431) (-2.2408, -15.4402) (-2.2386, -15.4494) (-2.2364, -15.4586) (-2.2342, -15.4679) (-2.232, -15.4772) (-2.2297, -15.4866) (-2.2274, -15.4959) (-2.2251, -15.5053) (-2.2228, -15.5147) (-2.2204, -15.5241) (-2.2181, -15.5336) (-2.2157, -15.5431) (-2.2133, -15.5526) (-2.2108, -15.5621) (-2.2084, -15.5716) (-2.2059, -15.5812) (-2.2034, -15.5908) (-2.2008, -15.6004) (-2.1983, -15.61) (-2.1957, -15.6197) (-2.1931, -15.6294) (-2.1905, -15.6391) (-2.1879, -15.6488) (-2.1852, -15.6585) (-2.1825, -15.6683) (-2.1798, -15.6781) (-2.1771, -15.6879) (-2.1743, -15.6978) (-2.1715, -15.7076) (-2.1687, -15.7175) (-2.1659, -15.7274) (-2.163, -15.7373) (-2.1602, -15.7473) (-2.1573, -15.7572) (-2.1543, -15.7672) (-2.1514, -15.7772) (-2.1484, -15.7872) (-2.1454, -15.7973) (-2.1424, -15.8074) (-2.1394, -15.8174) (-2.1363, -15.8275) (-2.1332, -15.8377) (-2.1307, -15.8458) (-2.1289, -15.8519) (-2.1276, -15.856) (-2.127, -15.858) knots 0 0 0 0 0 0 0.00416667 0.00833333 0.0125 0.01666667 0.02083333 0.025 0.02916667 0.03333333 0.0375 0.04166667 0.04583333 0.05 0.05416667 0.05833333 0.0625 0.06666667 0.07083333 0.075 0.07916667 0.08333333 0.0875 0.09166667 0.09583333 0.1 0.10416667 0.10833333 0.1125 0.11666667 0.12083333 0.125 0.12916667 0.13333333 0.1375 0.14166667 0.14583333 0.15 0.15416667 0.15833333 0.1625 0.16666667 0.17083333 0.175 0.17916667 0.18333333 0.1875 0.19166667 0.19583333 0.2 0.20416667 0.20833333 0.2125 0.21666667 0.22083333 0.225 0.22916667 0.23333333 0.2375 0.24166667 0.24583333 0.25 0.25416667 0.25833333 0.2625 0.26666667 0.27083333 0.275 0.27916667 0.28333333 0.2875 0.29166667 0.29583333 0.3 0.30416667 0.30833333 0.3125 0.31666667 0.32083333 0.325 0.32916667 0.33333333 0.3375 0.34166667 0.34583333 0.35 0.35416667 0.35833333 0.3625 0.36666667 0.37083333 0.375 0.37916667 0.38333333 0.3875 0.39166667 0.39583333 0.4 0.40416667 0.40833333 0.4125 0.41666667 0.42083333 0.425 0.42916667 0.43333333 0.4375 0.44166667 0.44583333 0.45 0.45416667 0.45833333 0.4625 0.46666667 0.47083333 0.475 0.47916667 0.48333333 0.4875 0.49166667 0.49583333 0.5 0.50416667 0.50833333 0.5125 0.51666667 0.52083333 0.525 0.52916667 0.53333333 0.5375 0.54166667 0.54583333 0.55 0.55416667 0.55833333 0.5625 0.56666667 0.57083333 0.575 0.57916667 0.58333333 0.5875 0.59166667 0.59583333 0.6 0.60416667 0.60833333 0.6125 0.61666667 0.62083333 0.625 0.62916667 0.63333333 0.6375 0.64166667 0.64583333 0.65 0.65416667 0.65833333 0.6625 0.66666667 0.67083333 0.675 0.67916667 0.68333333 0.6875 0.69166667 0.69583333 0.7 0.70416667 0.70833333 0.7125 0.71666667 0.72083333 0.725 0.72916667 0.73333333 0.7375 0.74166667 0.74583333 0.75 0.75416667 0.75833333 0.7625 0.76666667 0.77083333 0.775 0.77916667 0.78333333 0.7875 0.79166667 0.79583333 0.8 0.80416667 0.80833333 0.8125 0.81666667 0.82083333 0.825 0.82916667 0.83333333 0.8375 0.84166667 0.84583333 0.85 0.85416667 0.85833333 0.8625 0.86666667 0.87083333 0.875 0.87916667 0.88333333 0.8875 0.89166667 0.89583333 0.9 0.90416667 0.90833333 0.9125 0.91666667 0.92083333 0.925 0.92916667 0.93333333 0.9375 0.94166667 0.94583333 0.95 0.95416667 0.95833333 0.9625 0.96666667 0.97083333 0.975 0.97916667 0.98333333 0.9875 0.99166667 0.99583333 1 1 1 1 1 1
  arc A15 (-2.127, -15.858) -> (-1.2166, -15.9537) centre (0, 0) ccw
  spline S15 degree 5 poles (-1.2166, -15.9537) (-1.2155, -15.9518) (-1.2135, -15.9481) (-1.2104, -15.9425) (-1.2062, -15.9351) (-1.2011, -15.9258) (-1.196, -15.9166) (-1.1909, -15.9074) (-1.1859, -15.8981) (-1.1809, -15.8889) (-1.1759, -15.8797) (-1.1709, -15.8706) (-1.166, -15.8614) (-1.1611, -15.8523) (-1.1562, -15.8431) (-1.1514, -15.834) (-1.1465, -15.8249) (-1.1417, -15.8159) (-1.137, -15.8068) (-1.1322, -15.7977) (-1.1275, -15.7887) (-1.1228, -15.7797) (-1.1182, -15.7707) (-1.1135, -15.7617) (-1.1089, -15.7528) (-1.1043, -15.7438) (-1.0998, -15.7349) (-1.0952, -15.726) (-1.0907, -15.7171) (-1.0863, -15.7082) (-1.0818, -15.6993) (-1.0774, -15.6905) (-1.073, -15.6817) (-1.0687, -15.6729) (-1.0643, -15.6641) (-1.06, -15.6553) (-1.0557, -15.6466) (-1.0515, -15.6378) (-1.0472, -15.6291) (-1.043, -15.6204) (-1.0389, -15.6117) (-1.0347, -15.6031) (-1.0306, -15.5944) (-1.0265, -15.5858) (-1.0224, -15.5772) (-1.0184, -15.5686) (-1.0144, -15.5601) (-1.0104, -15.5515) (-1.0064, -15.543) (-1.0025, -15.5345) (-0.9986, -15.526) (-0.9947, -15.5176) (-0.9908, -15.5091) (-0.987, -15.5007) (-0.9832, -15.4923) (-0.9794, -15.484) (-0.9757, -15.4756) (-0.9719, -15.4673) (-0.9682, -15.459) (-0.9646, -15.4507) (-0.9609, -15.4424) (-0.9573, -15.4341) (-0.9537, -15.4259) (-0.9501, -15.4177) (-0.9466, -15.4095) (-0.9431, -15.4014) (-0.9396, -15.3932) (-0.9361, -15.3851) (-0.9327, -15.377) (-0.9293, -15.369) (-0.9259, -15.3609) (-0.9225, -15.3529) (-0.9192, -15.3449) (-0.9159, -15.3369) (-0.9126, -15.329) (-0.9094, -15.3211) (-0.9061, -15.3132) (-0.9029, -15.3053) (-0.8998, -15.2974) (-0.8966, -15.2896) (-0.8935, -15.2818) (-0.8904, -15.274) (-0.8873, -15.2663) (-0.8843, -15.2586) (-0.8812, -15.2509) (-0.8782, -15.2432) (-0.8753, -15.2355) (-0.8723, -15.2279) (-0.8694, -15.2203) (-0.8665, -15.2127) (-0.8636, -15.2052) (-0.8608, -15.1977) (-0.858, -15.1902) (-0.8552, -15.1827) (-0.8524, -15.1753) (-0.8497, -15.1679) (-0.8469, -15.1605) (-0.8442, -15.1531) (-0.8416, -15.1458) (-0.8389, -15.1385) (-0.8363, -15.1313) (-0.8337, -15.124) (-0.8311, -15.1168) (-0.8286, -15.1096) (-0.8261, -15.1025) (-0.8236, -15.0953) (-0.8211, -15.0882) (-0.8187, -15.0812) (-0.8162, -15.0741) (-0.8138, -15.0671) (-0.8115, -15.0601) (-0.8091, -15.0532) (-0.8068, -15.0463) (-0.8045, -15.0394) (-0.8022, -15.0325) (-0.8, -15.0257) (-0.7977, -15.0189) (-0.7955, -15.0122) (-0.7933, -15.0054) (-0.7912, -14.9987) (-0.789, -14.9921) (-0.7869, -14.9855) (-0.7848, -14.9789) (-0.7828, -14.9723) (-0.7807, -14.9658) (-0.7787, -14.9593) (-0.7767, -14.9528) (-0.7748, -14.9464) (-0.7728, -14.94) (-0.7709, -14.9336) (-0.769, -14.9273) (-0.7671, -14.921) (-0.7653, -14.9147) (-0.7634, -14.9085) (-0.7616, -14.9023) (-0.7599, -14.8961) (-0.7581, -14.89) (-0.7564, -14.8839) (-0.7546, -14.8779) (-0.7529, -14.8719) (-0.7513, -14.8659) (-0.7496, -14.86) (-0.748, -14.854) (-0.7464, -14.8482) (-0.7448, -14.8424) (-0.7433, -14.8366) (-0.7417, -14.8308) (-0.7402, -14.8251) (-0.7387, -14.8194) (-0.7372, -14.8138) (-0.7358, -14.8082) (-0.7344, -14.8027) (-0.733, -14.7971) (-0.7316, -14.7917) (-0.7302, -14.7862) (-0.7289, -14.7808) (-0.7276, -14.7755) (-0.7263, -14.7702) (-0.725, -14.7649) (-0.7237, -14.7597) (-0.7225, -14.7545) (-0.7213, -14.7493) (-0.7201, -14.7442) (-0.7189, -14.7392) (-0.7177, -14.7342) (-0.7166, -14.7292) (-0.7155, -14.7243) (-0.7144, -14.7194) (-0.7133, -14.7145) (-0.7123, -14.7097) (-0.7112, -14.705) (-0.7102, -14.7003) (-0.7092, -14.6956) (-0.7082, -14.691) (-0.7073, -14.6864) (-0.7064, -14.6819) (-0.7054, -14.6774) (-0.7045, -14.673) (-0.7037, -14.6686) (-0.7028, -14.6643) (-0.702, -14.66) (-0.7011, -14.6558) (-0.7003, -14.6516) (-0.6995, -14.6475) (-0.6988, -14.6434) (-0.698, -14.6394) (-0.6973, -14.6354) (-0.6966, -14.6314) (-0.6959, -14.6275) (-0.6952, -14.6237) (-0.6945, -14.6199) (-0.6939, -14.6162) (-0.6933, -14.6125) (-0.6926, -14.6089) (-0.6921, -14.6054) (-0.6915, -14.6018) (-0.6909, -14.5984) (-0.6904, -14.595) (-0.6898, -14.5916) (-0.6893, -14.5883) (-0.6888, -14.5851) (-0.6883, -14.5819) (-0.6879, -14.5788) (-0.6874, -14.5757) (-0.687, -14.5727) (-0.6866, -14.5698) (-0.6862, -14.5669) (-0.6858, -14.5641) (-0.6854, -14.5613) (-0.685, -14.5586) (-0.6847, -14.5559) (-0.6844, -14.5533) (-0.684, -14.5508) (-0.6837, -14.5484) (-0.6834, -14.546) (-0.6832, -14.5436) (-0.6829, -14.5414) (-0.6826, -14.5392) (-0.6824, -14.537) (-0.6822, -14.5349) (-0.6819, -14.5329) (-0.6817, -14.531) (-0.6815, -14.5291) (-0.6814, -14.5273) (-0.6812, -14.5256) (-0.681, -14.5239) (-0.6809, -14.5223) (-0.6807, -14.5208) (-0.6806, -14.5193) (-0.6805, -14.518) (-0.6804, -14.5167) (-0.6803, -14.5154) (-0.6802, -14.5143) (-0.6801, -14.5132) (-0.68, -14.5122) (-0.6799, -14.5112) (-0.6799, -14.5104) (-0.6798, -14.5096) (-0.6798, -14.5089) (-0.6797, -14.5083) (-0.6797, -14.5078) (-0.6797, -14.5074) (-0.6797, -14.5072) (-0.6796, -14.507) (-0.6796, -14.5069) knots -1 -1 -1 -1 -1 -1 -0.99583333 -0.99166667 -0.9875 -0.98333333 -0.97916667 -0.975 -0.97083333 -0.96666667 -0.9625 -0.95833333 -0.95416667 -0.95 -0.94583333 -0.94166667 -0.9375 -0.93333333 -0.92916667 -0.925 -0.92083333 -0.91666667 -0.9125 -0.90833333 -0.90416667 -0.9 -0.89583333 -0.89166667 -0.8875 -0.88333333 -0.87916667 -0.875 -0.87083333 -0.86666667 -0.8625 -0.85833333 -0.85416667 -0.85 -0.84583333 -0.84166667 -0.8375 -0.83333333 -0.82916667 -0.825 -0.82083333 -0.81666667 -0.8125 -0.80833333 -0.80416667 -0.8 -0.79583333 -0.79166667 -0.7875 -0.78333333 -0.77916667 -0.775 -0.77083333 -0.76666667 -0.7625 -0.75833333 -0.75416667 -0.75 -0.74583333 -0.74166667 -0.7375 -0.73333333 -0.72916667 -0.725 -0.72083333 -0.71666667 -0.7125 -0.70833333 -0.70416667 -0.7 -0.69583333 -0.69166667 -0.6875 -0.68333333 -0.67916667 -0.675 -0.67083333 -0.66666667 -0.6625 -0.65833333 -0.65416667 -0.65 -0.64583333 -0.64166667 -0.6375 -0.63333333 -0.62916667 -0.625 -0.62083333 -0.61666667 -0.6125 -0.60833333 -0.60416667 -0.6 -0.59583333 -0.59166667 -0.5875 -0.58333333 -0.57916667 -0.575 -0.57083333 -0.56666667 -0.5625 -0.55833333 -0.55416667 -0.55 -0.54583333 -0.54166667 -0.5375 -0.53333333 -0.52916667 -0.525 -0.52083333 -0.51666667 -0.5125 -0.50833333 -0.50416667 -0.5 -0.49583333 -0.49166667 -0.4875 -0.48333333 -0.47916667 -0.475 -0.47083333 -0.46666667 -0.4625 -0.45833333 -0.45416667 -0.45 -0.44583333 -0.44166667 -0.4375 -0.43333333 -0.42916667 -0.425 -0.42083333 -0.41666667 -0.4125 -0.40833333 -0.40416667 -0.4 -0.39583333 -0.39166667 -0.3875 -0.38333333 -0.37916667 -0.375 -0.37083333 -0.36666667 -0.3625 -0.35833333 -0.35416667 -0.35 -0.34583333 -0.34166667 -0.3375 -0.33333333 -0.32916667 -0.325 -0.32083333 -0.31666667 -0.3125 -0.30833333 -0.30416667 -0.3 -0.29583333 -0.29166667 -0.2875 -0.28333333 -0.27916667 -0.275 -0.27083333 -0.26666667 -0.2625 -0.25833333 -0.25416667 -0.25 -0.24583333 -0.24166667 -0.2375 -0.23333333 -0.22916667 -0.225 -0.22083333 -0.21666667 -0.2125 -0.20833333 -0.20416667 -0.2 -0.19583333 -0.19166667 -0.1875 -0.18333333 -0.17916667 -0.175 -0.17083333 -0.16666667 -0.1625 -0.15833333 -0.15416667 -0.15 -0.14583333 -0.14166667 -0.1375 -0.13333333 -0.12916667 -0.125 -0.12083333 -0.11666667 -0.1125 -0.10833333 -0.10416667 -0.1 -0.09583333 -0.09166667 -0.0875 -0.08333333 -0.07916667 -0.075 -0.07083333 -0.06666667 -0.0625 -0.05833333 -0.05416667 -0.05 -0.04583333 -0.04166667 -0.0375 -0.03333333 -0.02916667 -0.025 -0.02083333 -0.01666667 -0.0125 -0.00833333 -0.00416667 0 0 0 0 0 0
  line L30 (-0.6796, -14.5069) -> (-0.6796, -14.5063)
  line L31 (-0.6796, -14.5063) -> (-0.6435, -13.7349)
  arc A16 (-0.6435, -13.7349) -> (0.6435, -13.7349) centre (0, 0) ccw
  line L32 (0.6435, -13.7349) -> (0.6796, -14.5063)
  line L33 (0.6796, -14.5063) -> (0.6796, -14.5069)